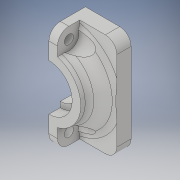
# Autodesk Inventor part: x-carriage-holder
Saved by Autodesk Inventor 2018 (Build 220112000, 112)
## iProperties
Created: 2017-10-14
Part Number: x-carriage-holder
Material: Generic
Document SubType Name: Modeling
Designer: Jurjen
Density: 1 g/cm^3
Appearance: Default
Author: Jurjen
Autodesk Inventor part; units mm, degrees
ref_plane "YZ Plane" through (0, 0, 0) normal (1, 0, 0) x (0, 1, 0)
ref_plane "XZ Plane" through (0, 0, 0) normal (0, 1, 0) x (-1, 0, 0)
ref_plane "XY Plane" through (0, 0, 0) normal (0, 0, 1) x (1, 0, 0)
sketch "Sketch1" plane through (0, 0, 0) normal (0, 0, 1) x (1, 0, 0)
  line L0 (0, 18.05) -> (16, 18.05)
  line L1 (16, 18.05) -> (16, -18.05)
  line L2 (16, -18.05) -> (0, -18.05)
  arc A0 (0, -8.15) -> (0, 8.15) centre (0, 0) ccw
  line L3 (0, -18.05) -> (0, -8.15)
  line L4 (0, 8.15) -> (0, 18.05)
  point P0 (16, 0)
  dimension "d0" = 16.3
  dimension "d1" = 36.1
  dimension "d3" = 16
  constraints: 10 end point, 3 parallel, 2 point on circle, 2 vertical alignment, 1 centre point, 1 coincident, 1 horizontal, 1 horizontal alignment, 1 midpoint, 1 perpendicular
  measures "d0" diameter of A0
  measures "d1" distance of L2.end L0.start
  measures "d3" distance between parallel lines of L1 L4
extrude "Extrusion1" add sketch "Sketch1" along normal mid plane 5
sketch "Sketch2" plane through (0, 0, 2.5) normal (0, 0, 1) x (1, 0, 0)
  arc A0 (0, -6.25) -> (0, 6.25) centre (0, 0) ccw
  arc A1 (0, -8.15) -> (0, 8.15) centre (0, 0) ccw
  line L0 (0, 6.25) -> (0, 8.15)
  line L1 (0, -6.25) -> (0, -8.15)
  dimension "d6" = 12.5
  constraints: 4 end point, 4 point on circle, 2 centre point, 2 coincident, 2 vertical
  measures "d6" diameter of A0
extrude "Extrusion2" add sketch "Sketch2" along normal blind 3.8 and the other way blind 1.8
sketch "Sketch3" plane through (0, 0, 6.3) normal (0, 0, 1) x (1, 0, 0)
  arc A0 (0, -8.15) -> (0, 8.15) centre (0, 0) ccw projected
  arc A1 (0, -11.15) -> (0, 11.15) centre (0, 0) ccw
  line L0 (0, -8.15) -> (0, -11.15)
  line L1 (0, 8.15) -> (0, 11.15)
  dimension "d11" = 3
  constraints: 4 end point, 3 point on circle, 1 centre point, 1 coincident, 1 vertical
  measures "d11" radial gap between concentric circles of A1 A0
extrude "Extrusion3" add sketch "Sketch3" along normal blind 4
sketch "Sketch4" plane through (0, 0, 6.3) normal (0, 0, -1) x (-1, 0, 0)
  arc A0 (0, 8.15) -> (0, -8.15) centre (0, 0) ccw projected
  line L0 (0, 11.15) -> (0, 8.15) projected
  arc A1 (0, 11.15) -> (0, -11.15) centre (0, 0) ccw projected
  line L1 (0, -8.15) -> (0, -11.15) projected
extrude "Extrusion4" add sketch "Sketch4" along normal up to surface (3.8 mm away)
sketch "Sketch5" plane through (0, 0, 2.5) normal (0, 0, 1) x (1, 0, 0)
  arc A0 (0, -11.15) -> (0, 11.15) centre (0, 0) ccw projected
  line L0 (16, 18.05) -> (0, 18.05) projected
  line L1 (3, 18.05) -> (3, 10.7388)
  arc A1 (0, -11.15) -> (0, 11.15) centre (0, 0) ccw projected
  line L2 (3, -10.7388) -> (3, -18.05)
  line L3 (0, -18.05) -> (16, -18.05) projected
  line L4 (0, 18.05) -> (0, 11.15) projected
  line L5 (0, -11.15) -> (0, -18.05) projected
  dimension "d16" = 3
  constraints: 4 end point, 4 point on line, 2 point on circle, 1 vertical
  measures "d16" distance between parallel lines of L4 L1
extrude "Extrusion5" add sketch "Sketch5" along normal up to surface (7.8 mm away)
chamfer "Chamfer1" distance 5 angle 45 1 edges at (11.15, 0, 2.5)
fillet "Fillet1" radius 3 3 edges at (11.7041, -11.1281, 2.5) (11.15, 0, 7.5) (11.7041, 11.1281, 2.5)
sketch "Sketch6" plane through (3, -18.05, 2.5) normal (1, 0, 0) x (0, 0, -1)
  circle A0 centre (-3.8, 32.1) radius 1.6
  circle A1 centre (-3.8, 4) radius 1.6
  line L0 (0, 0) -> (-7.8, 0) projected
  line L1 (-7.8, 7.3112) -> (-7.8, 0) projected
  line L2 (0, 36.1) -> (-7.8, 36.1) projected
  point P0 (2.5, 18.05)
  dimension "d19" = 3.2
  dimension "d20" = 4
  dimension "d21" = 4
  dimension "d22" = 4
  constraints: 2 centre point, 1 equal radius, 1 vertical alignment
  measures "d19" diameter of A1
  measures "d20" distance from line of A1.centre L0
  measures "d21" distance from line of A1.centre L1
  measures "d22" distance from line of L2 A0.centre
extrude "Extrusion6" cut sketch "Sketch6" against normal up to next
fillet "Fillet2" radius 4 2 edges at (1.5, -18.05, 10.3) (1.5, 18.05, 10.3)
fillet "Fillet3" radius 4 2 edges at (16, -18.05, 0) (16, 18.05, 0)
sketch "Sketch7" plane through (3, -18.05, 2.5) normal (1, 0, 0) x (0, 0, -1)
  arc A0 (-3.2482, 5.5018) -> (-2.2844, 4.5129) centre (-3.8, 4) ccw projected
  arc A1 (-2.2844, 31.5871) -> (-3.2482, 30.5982) centre (-3.8, 32.1) ccw projected
  circle A2 centre (-3.8, 4) radius 3.5
  circle A3 centre (-3.8, 32.1) radius 3.5
  point P0 (2.5, 18.05)
  dimension "d31" = 7
  constraints: 2 centre point, 2 coincident, 1 equal radius
  measures "d31" diameter of A2
extrude "Extrusion7" cut sketch "Sketch7" along normal through all
body "Solid1"
